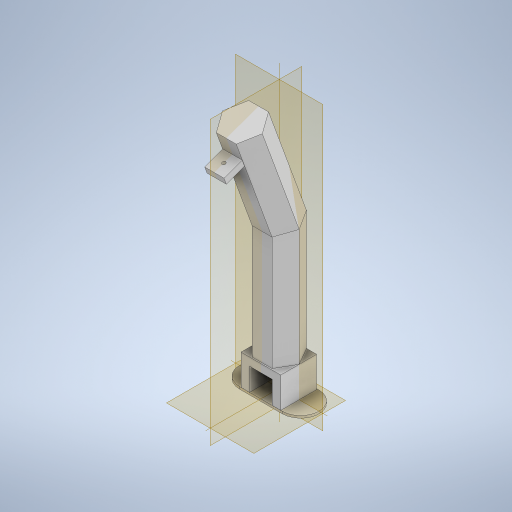
# Autodesk Inventor part: Kamerahalter_II
Saved by Autodesk Inventor 2023 (Build 270158000, 158)
## iProperties
Created: 2022-07-05
Part Number: Kamerahalter_II
Material: Generic
Document SubType Name: Modeling
Designer: Habib
Density: 1 g/cm^3
Appearance: Default
Author: Habib
Autodesk Inventor part; units mm, degrees
sketch "Sketch1" plane through (0, 0, 0) normal (0, 1, 0) x (-1, 0, 0)
  line L0 (0, 0) -> (17.5, 0)
  line L1 (17.5, 0) -> (8.75, -15.1554)
  line L2 (8.75, -15.1554) -> (-8.75, -15.1554)
  line L3 (-8.75, -15.1554) -> (-17.5, 0)
  line L4 (-17.5, 0) -> (-8.75, 15.1554)
  line L5 (-8.75, 15.1554) -> (8.75, 15.1554)
  line L6 (8.75, 15.1554) -> (17.5, 0)
  dimension "d1" = 17.5
  constraints: 14 end point, 1 coincident, 1 horizontal, 13 other
  measures "d1" distance of L0.start L0.end
sketch "Sketch3" plane through (0, 0, 0) normal (1, 0, 0) x (0, 1, 0)
  line L0 (0, 0) -> (130, 0)
  line L1 (130, 0) -> (219.2708, 32.4919)
  dimension "d5" = 130
  dimension "d6" = 95
  dimension "d7" = 160
  constraints: 4 end point, 1 horizontal
  measures "d5" distance of L0.start L0.end
  measures "d6" distance of L0.end L1.end
  measures "d7" angle of L1 L0
sweep "Sweep1" add profiles "Sketch1" path "Sketch3"
sketch "Sketch4" plane through (-8.75, 127.3277, 15.1554) normal (0, -0.3420201, 0.9396926) x (1, 0, 0)
  line L0 (0, 92.3277) -> (17.5, 92.3277) projected
  line L1 (8.75, 92.3277) -> (8.75, 76.3277)
  line L2 (8.75, 76.3277) -> (17.25, 76.3277)
  line L3 (17.5, 0) -> (17.5, 92.3277) projected
  line L4 (17.25, 76.3277) -> (17.25, 70.3277)
  line L5 (17.25, 70.3277) -> (0.25, 70.3277)
  line L6 (0, 0) -> (0, 92.3277) projected
  line L7 (0.25, 70.3277) -> (0.25, 76.3277)
  line L8 (0.25, 76.3277) -> (8.75, 76.3277)
  point P0 (8.75, -124.8324)
  dimension "d10" = 16
  dimension "d11" = 8.5
  dimension "d12" = 6
  dimension "d13" = 17
  constraints: 12 end point, 5 perpendicular, 1 midpoint, 1 point on line, 1 vertical
  measures "d10" distance of L1.start L1.end
  measures "d11" distance of L1.end L2.end
  measures "d12" distance of L2.end L4.end
  measures "d13" distance of L4.end L5.end
extrude "Extrusion1" add sketch "Sketch4" along normal blind 17
sketch "Sketch5" plane through (-8.5, 199.0522, 41.2611) normal (0, 0.9396926, 0.3420201) x (1, 0, 0)
  line L0 (17, 0) -> (0, 0) projected
  line L1 (8.5, 0) -> (8.5, -8)
  circle A0 centre (8.5, -8) radius 2.5
  point P0 (8.5, -29.3072)
  dimension "d16" = 8
  dimension "d17" = 5
  constraints: 2 end point, 1 centre point, 1 coincident, 1 midpoint, 1 vertical
  measures "d16" distance of L1.start L1.end
  measures "d17" diameter of A0
hole "Hole1" at (0, 196.3161, 48.7786) direction (0, -0.9396926, -0.3420201) diameter 3 depth 10.077 tip angle 118
sketch "Sketch6" plane through (0, 0, 0) normal (0, 1, 0) x (-1, 0, 0)
  line L0 (17.5, 0) -> (8.75, 15.1554) projected
  line L1 (17.5, 0) -> (17.5, -15.4226)
  line L2 (17.5, -15.4226) -> (-17.5, -15.4226)
  line L3 (-17.5, -15.4226) -> (-17.5, 16.246)
  line L4 (-17.5, 0) -> (-17.5, 32.4919) projected
  line L5 (17.5, 0) -> (17.5, 32.4919) projected
  line L6 (17.5, 16.246) -> (-17.5, 16.246)
  line L7 (17.5, 16.246) -> (17.5, 0)
  point P0 (0, 0)
  constraints: 10 end point, 3 perpendicular, 2 midpoint, 1 vertical
extrude "Extrusion2" add sketch "Sketch6" along normal blind 27
sketch "Sketch7" plane through (-17.5, 0, 16.246) normal (0, 0, 1) x (1, 0, 0)
  line L0 (17.5, 0) -> (7.5, 0)
  line L1 (35, 0) -> (0, 0) projected
  line L2 (7.5, 0) -> (27.5, 0)
  line L3 (7.5, 0) -> (7.5, 20)
  line L4 (7.5, 20) -> (27.5, 20)
  line L5 (27.5, 20) -> (27.5, 0)
  dimension "d27" = 10
  dimension "d28" = 20
  dimension "d29" = 20
  constraints: 10 end point, 2 perpendicular, 2 point on line, 1 vertical
  measures "d27" distance of L0.start L0.end
  measures "d28" distance of L0.end L2.end
  measures "d29" distance of L0.end L3.end
extrude "Extrusion3" cut sketch "Sketch7" against normal blind 50
sketch "Sketch8" plane through (0, 0, 0) normal (0, 1, 0) x (-1, 0, 0)
  line L0 (0, 0) -> (-35, 0)
  line L1 (-35, 0) -> (35, 0) construction
  line L2 (-18.8264, -16.1736) -> (18.8264, -16.1736)
  line L3 (18.8264, 16.1736) -> (-18.8264, 16.1736)
  arc A0 (-18.8264, 16.1736) -> (-18.8264, -16.1736) centre (-18.8264, 0) ccw
  arc A1 (18.8264, -16.1736) -> (18.8264, 16.1736) centre (18.8264, 0) ccw
  dimension "d32" = 35
  dimension "d33" = 70
  constraints: 10 end point, 6 point on circle, 4 tangent, 3 point on line, 2 centre point, 1 horizontal, 1 midpoint, 1 parallel
  measures "d32" distance of L0.start L0.end
  measures "d33" distance of L0.end L1.end
extrude "Extrusion4" add sketch "Sketch8" against normal blind 2
body "Solid1"
